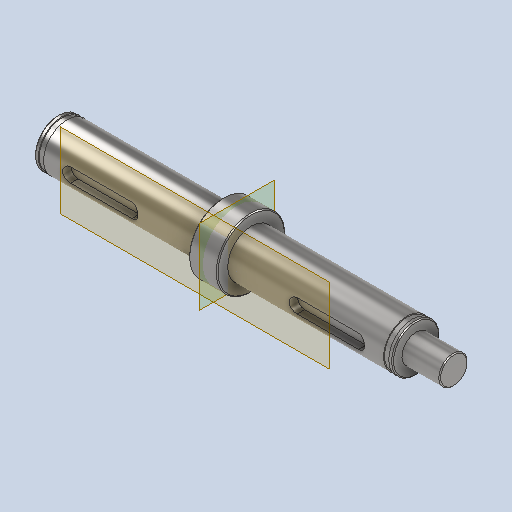
# Autodesk Inventor part: ParallelSystem_ProximalPart_Shaft_Driven
Saved by Autodesk Inventor 2022 (Build 260153000, 153)
## iProperties
Created: 2022-07-19
Part Number: ParallelSystem_ProximalPart_Shaft_Driven
Material: Edelstahl
Document SubType Name: Modeling
Designer: alexw
Density: 8 g/cm^3
Appearance: Halbpoliert
Mass: 32.905 g
Surface Area: 19.9344 cm^2
Volume: 4.11312 cm^3
ParrallelMecha_DrivenLink_OuterWidth: 72,000 mm
Querstrebe_Length: 44,000 mm
Author: alexw
Autodesk Inventor part; units mm, degrees
ref_plane "YZ Plane" through (0, 0, 0) normal (1, 0, 0) x (0, 1, 0)
ref_plane "XZ Plane" through (0, 0, 0) normal (0, 1, 0) x (-1, 0, 0)
sketch "Skizze1" plane through (0, 0, 0) normal (0, 0, 1) x (1, 0, 0)
  line L0 (0, 0) -> (0, 5)
  line L1 (0, 5) -> (0.8, 5)
  line L2 (0.8, 5) -> (0.8, 4.8)
  line L3 (0.8, 4.8) -> (1.9, 4.8)
  line L4 (1.9, 4.8) -> (1.9, 5)
  line L5 (1.9, 5) -> (34.9, 5)
  line L6 (34.9, 5) -> (34.9, 7.25)
  line L7 (34.9, 7.25) -> (40.9, 7.25)
  line L8 (40.9, 7.25) -> (40.9, 5)
  line L9 (40.9, 5) -> (73.9, 5)
  line L10 (73.9, 5) -> (73.9, 4.8)
  line L11 (73.9, 4.8) -> (75, 4.8)
  line L12 (75, 4.8) -> (75, 5)
  line L13 (75, 5) -> (75.8, 5)
  line L14 (75.8, 5) -> (75.8, 3)
  line L15 (75.8, 3) -> (83.8, 3)
  line L16 (83.8, 3) -> (83.8, 0)
  line L17 (83.8, 0) -> (0, 0)
  line L18 (25.9, 5) -> (25.9, 0) construction
  line L19 (49.9, 5) -> (49.9, 0) construction
  line L20 (15.9, 5) -> (15.9, 0) construction
  line L21 (59.9, 5) -> (59.9, 0) construction
  dimension "d0" = 10
  dimension "d1" = 6
  dimension "d2" = 14.5
  dimension "d3" = 1.1
  dimension "d4" = 9.6
  dimension "d5" = 0.8
  dimension "d6" = 0.8
  dimension "d7" = 9
  dimension "d8" = 9
  dimension "d9" = 6
  dimension "d10" = 24
  dimension "d11" = 24
  dimension "d12" = 8
  dimension "ParrallelMecha_DrivenLink_OuterWidth" = 72
  dimension "d22" = 10
  dimension "d23" = 10
  dimension "Querstrebe_Length" = 44
  constraints: 44 end point, 18 perpendicular, 14 point on line, 2 collinear, 1 vertical
  measures "d0" diameter of L5 L17
  measures "d1" diameter of L15 L17
  measures "d2" diameter of L7 L17
  measures "d3" distance of L3.end L2.end
  measures "d4" diameter of L3 L17
  measures "d5" distance between parallel lines of L2 L0
  measures "d6" distance between parallel lines of L14 L12
  measures "d7" distance between parallel lines of L6 L18
  measures "d8" distance between parallel lines of L8 L19
  measures "d9" distance between parallel lines of L8 L6
  measures "d10" distance between parallel lines of L4 L18
  measures "d11" distance between parallel lines of L19 L10
  measures "d12" distance between parallel lines of L14 L16
  measures "ParrallelMecha_DrivenLink_OuterWidth" distance between parallel lines of L10 L4
  measures "d22" distance between parallel lines of L19 L21
  measures "d23" distance between parallel lines of L20 L18
  measures "Querstrebe_Length" distance between parallel lines of L21 L20
revolve "Umdrehung1" add sketch "Skizze1" angle 360 about axis through (83.8, 0, 0) along (-1, 0, 0)
chamfer "Fase1" distance 0.2 angle 45 5 edges at (34.9, -7.25, 0) (40.9, -7.25, 0) (75.8, -5, 0) (83.8, -3, 0) (0, -5, 0)
ref_plane "Wellennut_Spiegelebene" through (37.9, 0, 0) normal (-1, 0, 0) x (0, 0, 1)
ref_plane "Arbeitsebene2" through (18.4, 0, 5) normal (0, 0, 1) x (1, 0, 0)
sketch "Skizze3" plane through (18.4, 0, 5) normal (0, 0, 1) x (1, 0, 0)
  line L0 (7.5, 5) -> (7.5, 0) construction
  line L1 (-35.16, 0) -> (82.16, 0) construction
  line L2 (2, 0) -> (-11, 0) construction
  line L3 (2, 1.5) -> (-11, 1.5)
  line L4 (-11, -1.5) -> (2, -1.5)
  arc A0 (2, -1.5) -> (2, 1.5) centre (2, 0) ccw
  arc A1 (-11, 1.5) -> (-11, -1.5) centre (-11, 0) ccw
  line L5 (-16.5, 0) -> (7.5, 0) construction
  line L6 (-16.5, -5) -> (-16.5, 5) construction
  point P0 (-18.4, 0)
  point P1 (-4.5, 0)
  point P2 (-4.5, 0)
  dimension "d17" = 3
  dimension "d18" = 16
  constraints: 10 end point, 4 point on circle, 4 tangent, 3 midpoint, 2 centre point, 2 horizontal, 2 point on line, 1 coincident, 1 collinear, 1 parallel
  measures "d17" distance between parallel lines of L4 L3
extrude "Wellennut" cut sketch "Skizze3" against normal blind 1.8
mirror "Spiegeln1" about plane through (37.9, 0, 0) normal (-1, 0, 0) of "Wellennut"
equation "\"d10\" = ParallelLink_Lever_Thickness_1 + ParallelLink_BearingStep_Height_1"
equation "\"d11\" = d10"
equation "\"d22\" = ParallelLink_BearingStep_Height_1"
equation "\"d23\" = d22"
equation "\"ParallelLink_Lever_Thickness_1\" = 14"
equation "\"ParallelLink_BearingStep_Height_1\" = 10"
